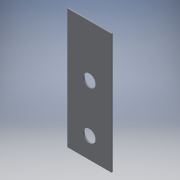
# Autodesk Inventor part: L plate
Saved by Autodesk Inventor 2018 (Build 220112000, 112)
## iProperties
Created: 2018-01-23
Part Number: L plate
Material: Generic
Document SubType Name: Modeling
Designer: jahu2
Density: 1 g/cm^3
Appearance: Default
Author: jahu2
Autodesk Inventor part; units mm, degrees
ref_plane "YZ Plane" through (0, 0, 0) normal (1, 0, 0) x (0, 1, 0)
ref_plane "XZ Plane" through (0, 0, 0) normal (0, 1, 0) x (-1, 0, 0)
ref_plane "XY Plane" through (0, 0, 0) normal (0, 0, 1) x (1, 0, 0)
sketch "Sketch1" plane through (0, 0, 0) normal (0, 0, 1) x (1, 0, 0)
  line L0 (0, 0) -> (-101.6, 0)
  line L1 (-101.6, 0) -> (-101.6, -276.225)
  line L2 (-101.6, -276.225) -> (0, -276.225)
  line L3 (0, -276.225) -> (0, 0)
  circle A0 centre (-50.8, -228.6) radius 14.2875
  circle A1 centre (-50.8, -118.5672) radius 14.2875
  dimension "d0" = 101.6
  dimension "d1" = 276.225
  dimension "d2" = 28.575
  dimension "d3" = 110.0328
  dimension "d4" = 28.575
  dimension "d5" = 50.8
  dimension "d6" = 47.625
  dimension "d7" = 50.8
  constraints: 8 end point, 2 centre point, 2 parallel, 1 horizontal, 1 perpendicular
  measures "d0" distance of L2.end L1.end
  measures "d1" distance of L1.end L0.end
  measures "d2" diameter of A1
  measures "d3" distance of A0.centre A1.centre
  measures "d4" diameter of A0
  measures "d5" distance from line of L1 A0.centre
  measures "d6" distance from line of L2 A0.centre
  measures "d7" distance from line of L1 A1.centre
extrude "Extrusion1" add sketch "Sketch1" along normal blind 3.175
body "Solid1"
